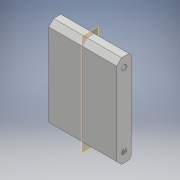
# Autodesk Inventor part: Chassis
Saved by Autodesk Inventor 2018 (Build 220112000, 112)
## iProperties
Created: 2018-04-07
Part Number: Chassis
Material: Générique
Document SubType Name: Modeling
Designer: Dimitri
Density: 1 g/cm^3
Appearance: Par défaut
Author: Dimitri
Autodesk Inventor part; units mm, degrees
ref_plane "YZ Plane" through (0, 0, 0) normal (1, 0, 0) x (0, 1, 0)
ref_plane "XZ Plane" through (0, 0, 0) normal (0, 1, 0) x (-1, 0, 0)
ref_plane "XY Plane" through (0, 0, 0) normal (0, 0, 1) x (1, 0, 0)
sketch "Esquisse1" plane through (0, 0, 0) normal (0, 1, 0) x (-1, 0, 0)
  line L0 (-70, 95) -> (70, 95)
  line L1 (70, 95) -> (70, -95)
  line L2 (70, -95) -> (-70, -95)
  line L3 (-70, -95) -> (-70, 95)
  line L4 (-70, 95) -> (70, -95) construction
  line L5 (70, 95) -> (-70, -95) construction
  point P0 (0, 0)
  dimension "d0" = 140
  dimension "d1" = 190
  constraints: 12 end point, 2 midpoint, 2 parallel, 1 horizontal, 1 perpendicular
  measures "d0" distance of L1.end L2.end
  measures "d1" distance of L0.end L1.end
extrude "Extrusion1" add sketch "Esquisse1" along normal blind 30
chamfer "Chanfrein1" distance 10 angle 45 2 edges at (0, 0, 95) (0, 0, -95)
chamfer "Chanfrein2" distance 5 angle 45 2 edges at (0, 30, 95) (0, 30, -95)
shell "Coque1" thickness 2 removed faces 1 at (23.3333, 30, 30)
sketch "Esquisse2" plane through (70, 0, 85) normal (1, 0, 0) x (0, 0, -1)
  line L0 (-10, 10) -> (-10, 25) projected
  line L1 (180, 10) -> (180, 25) projected
  line L2 (-5, 30) -> (175, 30) projected
  line L3 (170, 0) -> (0, 0) projected
  circle A0 centre (10, 15) radius 5
  line L4 (85, 0) -> (85, 30)
  circle A1 centre (160, 15) radius 5
  dimension "d11" = 10
  dimension "d12" = 20
  dimension "d13" = 15
  constraints: 2 centre point, 2 end point, 1 midpoint, 1 symmetric about line, 1 other
  measures "d11" diameter of A0
  measures "d12" distance from line of L0 A0.centre
  measures "d13" distance from line of L3 A0.centre
extrude "Extrusion2" cut sketch "Esquisse2" against normal blind 3
ref_plane "Plan de construction1" through (0, 0, 85) normal (1, 0, 0) x (0, 0, -1)
mirror "Symétrie1" about plane through (0, 0, 85) normal (1, 0, 0) of "Extrusion2"
